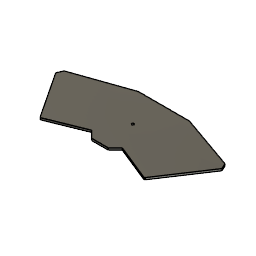
jianpanke (Autodesk Fusion 360 design; units mm, degrees)
part number: 2026-01-06-10-14-55-498
Autodesk Fusion 360 part; units mm, degrees
sketch "Sketch1" plane through (0, 0, 0) normal (0, 0, 1) x (1, 0, 0)
  line L0 (0, 0) -> (0, 100)
  line L1 (0, 0) -> (-13, 0)
  line L2 (-13, 0) -> (-23.9602, 10.9602)
  line L3 (-13, 0) -> (2.5, 0) construction
  line L4 (-23.9602, 10.9602) -> (-80.982, -12.0782)
  line L5 (-23.9602, 10.9602) -> (37.5398, 10.9602) construction
  line L6 (-80.982, -12.0782) -> (-82.2107, -11.2178)
  line L7 (-80.982, -12.0782) -> (-79.482, -12.0782) construction
  line L8 (-82.2107, -11.2178) -> (-129.9532, 60.9133)
  line L9 (-82.2107, -11.2178) -> (4.2893, -11.2178) construction
  line L10 (-129.9532, 60.9133) -> (-125.7271, 69.9764)
  line L11 (-129.9532, 60.9133) -> (-119.9532, 60.9133) construction
  line L12 (-125.7271, 69.9764) -> (-40, 100)
  line L13 (-40, 100) -> (0, 100)
  line L14 (13, 0) -> (-2.5, 0) construction
  line L15 (13, 0) -> (23.9602, 10.9602)
  line L16 (23.9602, 10.9602) -> (80.982, -12.0782)
  line L17 (82.2107, -11.2178) -> (129.9532, 60.9133)
  line L18 (80.982, -12.0782) -> (82.2107, -11.2178)
  line L19 (129.9532, 60.9133) -> (125.7271, 69.9764)
  line L20 (125.7271, 69.9764) -> (40, 100)
  line L21 (40, 100) -> (0, 100)
  line L22 (13, 0) -> (0, 0)
  dimension "d1" = 100
  dimension "d2" = 13
  dimension "d3" = 135
  dimension "d4" = 15.5
  dimension "d5" = 158
  dimension "d6" = 61.5
  dimension "d7" = 145
  dimension "d8" = 1.5
  dimension "d9" = 123.5
  dimension "d10" = 86.5
  dimension "d11" = 65
  dimension "d12" = 10
  constraint coincident L0.start L1.start
  constraint vertical L0
  constraint perpendicular L0 L1
  constraint horizontal L3
  constraint horizontal L5
  constraint horizontal L7
  constraint horizontal L9
  constraint horizontal L11
  constraint perpendicular L0 L13
  constraint symmetric L13.end L0 L21.end
  constraint symmetric L0 L1.end L14.start
  constraint symmetric L0 L2.end L15.end
  constraint symmetric L0 L3.end L14.end
  constraint symmetric L0 L4.end L16.end
  constraint symmetric L0 L6.end L17.start
  constraint symmetric L0 L8.end L17.end
  constraint symmetric L0 L10.end L19.end
  constraint symmetric L0 L12.end L20.end
  measures "d1" distance of L0.start L0.end
  measures "d2" distance of L0.start L1.end
  measures "d3" angle of L2 L3
  measures "d4" distance of L1.end L2.end
  measures "d5" angle of L4 L5
  measures "d6" distance of L2.end L4.end
  measures "d7" angle of L6 L7
  measures "d8" distance of L4.end L6.end
  measures "d9" angle of L8 L9
  measures "d10" distance of L6.end L8.end
  measures "d11" angle of L10 L11
  measures "d12" distance of L8.end L10.end
extrude "Extrude1" add sketch "Sketch1" along normal blind 3
sketch "Sketch2" plane through (0, 0, 3) normal (0, 0, 1) x (-1, 0, 0)
  line L0 (-23.9602, -10.9602) -> (-80.982, 12.0782)
  line L1 (-80.982, 12.0782) -> (-82.2107, 11.2178)
  line L2 (-82.2107, 11.2178) -> (-129.9532, -60.9133)
  line L3 (-129.9532, -60.9133) -> (-125.7271, -69.9764)
  line L4 (-125.7271, -69.9764) -> (-40, -100)
  line L5 (-40, -100) -> (40, -100)
  line L6 (40, -100) -> (125.7271, -69.9764)
  line L7 (125.7271, -69.9764) -> (129.9532, -60.9133)
  line L8 (129.9532, -60.9133) -> (82.2107, 11.2178)
  line L9 (82.2107, 11.2178) -> (80.982, 12.0782)
  line L10 (80.982, 12.0782) -> (23.9602, -10.9602)
  line L11 (23.9602, -10.9602) -> (13, 0)
  line L12 (13, 0) -> (-13, 0)
  line L13 (-13, 0) -> (-23.9602, -10.9602)
  line L14 (0, 0) -> (0, -51.5)
  circle A0 centre (0, -51.5) radius 1.75
  dimension "d15" = 51.5
  dimension "d16" = 3.5
  constraint coincident L14.start origin
  constraint perpendicular L12 L14
  constraint coincident L14.end A0.centre
  measures "d15" distance of L14.start L14.end
  measures "d16" diameter of A0
extrude "Extrude2" cut sketch "Sketch2" against normal up to surface (3 mm away) contours A0
